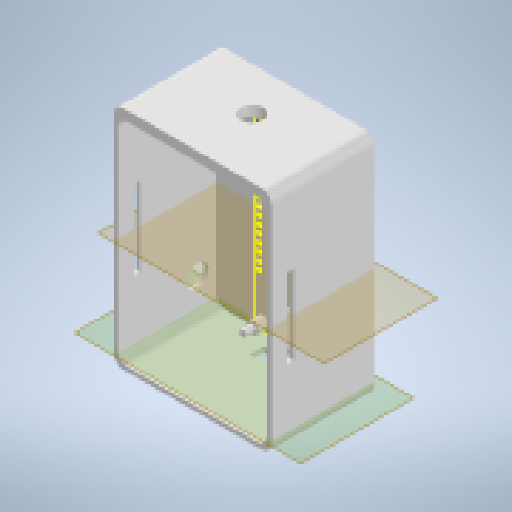
# Autodesk Inventor part: Casev2
Saved by Autodesk Inventor 2025.2 (Build 292293000, 293)
## iProperties
Created: 2022-04-07
Part Number: Casev2
Material: Generic
Document SubType Name: Modeling
Designer: Fred
Density: 1 g/cm^3
Appearance: Default
Author: Fred
## iProperties of the stored document CaseV2_3DPrint.ipt
Created: 2022-04-13
Part Number: CaseV2_3DPrint
Material: Generic
Document SubType Name: Modeling
Designer: Fred
Density: 1 g/cm^3
Appearance: Default
Author: Fred
Autodesk Inventor part; units mm, degrees
ref_plane "YZ Plane" through (0, 0, 0) normal (1, 0, 0) x (0, 1, 0)
ref_plane "XZ Plane" through (0, 0, 0) normal (0, 1, 0) x (-1, 0, 0)
sketch "Sketch1" plane through (0, 0, 0) normal (0, 0, 1) x (1, 0, 0)
  line L0 (0, 0) -> (50.8, 0)
  line L1 (50.8, 0) -> (50.8, 71.12)
  line L2 (50.8, 71.12) -> (0, 71.12)
  line L3 (0, 71.12) -> (0, 0)
  dimension "d0" = 71.12
  dimension "d1" = 50.8
  constraints: 8 end point, 2 parallel, 1 horizontal, 1 perpendicular
  measures "d0" distance of L0.end L1.end
  measures "d1" distance of L1.end L2.end
extrude "Extrusion1" add sketch "Sketch1" along normal blind 33
shell "Shell1" thickness 1.5 removed faces 1 at (33.8667, 23.7067, 33)
sketch "Sketch5" plane through (1.5, 69.62, 1.5) normal (0, 0, 1) x (1, 0, 0)
  circle A0 centre (15.01, -10.335) radius 1.1 projected
  circle A1 centre (15.01, -65.58) radius 1.25 projected
  circle A2 centre (32.79, -65.58) radius 1.25 projected
  circle A3 centre (13.74, -31.29) radius 0.6352 projected
  circle A4 centre (13.74, -23.67) radius 0.6352 projected
  circle A5 centre (34.06, -38.91) radius 0.6352 projected
  circle A6 centre (34.06, -41.45) radius 0.6352 projected
  circle A7 centre (34.06, -59.23) radius 0.6352 projected
  circle A8 centre (18.185, -32.544) radius 0.501 projected
  circle A9 centre (34.06, -31.29) radius 0.6352 projected
  circle A10 centre (13.74, -38.91) radius 0.6352 projected
  circle A11 centre (34.06, -54.15) radius 0.6352 projected
  circle A12 centre (34.06, -49.07) radius 0.6352 projected
  circle A13 centre (34.06, -23.67) radius 0.6352 projected
  circle A14 centre (13.74, -41.45) radius 0.6352 projected
  circle A15 centre (34.06, -28.75) radius 0.6352 projected
  circle A16 centre (13.74, -28.75) radius 0.6352 projected
  circle A17 centre (34.06, -26.21) radius 0.6352 projected
  circle A18 centre (34.06, -61.77) radius 0.6352 projected
  circle A19 centre (13.74, -51.61) radius 0.6352 projected
  circle A20 centre (34.06, -51.61) radius 0.6352 projected
  circle A21 centre (13.74, -49.07) radius 0.6352 projected
  circle A22 centre (34.06, -36.37) radius 0.6352 projected
  circle A23 centre (34.06, -46.53) radius 0.6352 projected
  circle A24 centre (34.06, -56.69) radius 0.6352 projected
  circle A25 centre (20.217, -30.544) radius 0.501 projected
  circle A26 centre (15.01, -10.335) radius 1.1 projected
  circle A27 centre (15.01, -65.58) radius 1.25 projected
  circle A28 centre (32.79, -65.58) radius 1.25 projected
  circle A29 centre (18.185, -30.544) radius 0.501 projected
  circle A30 centre (20.217, -32.544) radius 0.501 projected
  circle A31 centre (13.74, -36.37) radius 0.6352 projected
  circle A32 centre (34.06, -43.99) radius 0.6352 projected
  circle A33 centre (13.74, -33.83) radius 0.6352 projected
  circle A34 centre (13.74, -26.21) radius 0.6352 projected
  circle A35 centre (13.74, -46.53) radius 0.6352 projected
  circle A36 centre (34.06, -33.83) radius 0.6352 projected
  circle A37 centre (13.74, -43.99) radius 0.6352 projected
  line L0 (21.233, -68.12) -> (21.741, -67.612) projected
  line L1 (21.741, -67.612) -> (25.932, -67.612) projected
  line L2 (25.932, -67.612) -> (26.44, -68.12) projected
  line L3 (26.44, -68.12) -> (32.79, -68.12) projected
  arc A38 (32.79, -68.12) -> (35.33, -65.58) centre (32.79, -65.58) ccw projected
  line L4 (35.33, -65.58) -> (35.33, -10.335) projected
  arc A39 (35.33, -10.335) -> (32.79, -7.795) centre (32.79, -10.335) ccw projected
  line L5 (32.79, -7.795) -> (15.01, -7.795) projected
  arc A40 (15.01, -7.795) -> (12.47, -10.335) centre (15.01, -10.335) ccw projected
  line L6 (12.47, -10.335) -> (12.47, -65.58) projected
  arc A41 (12.47, -65.58) -> (15.01, -68.12) centre (15.01, -65.58) ccw projected
  line L7 (15.01, -68.12) -> (21.233, -68.12) projected
  point P0 (-1.5, -69.62)
  constraints: 3 coincident
ref_plane "Work Plane2" through (16.51, 4.04, 1.5) normal (0, -1, 0) x (1, 0, 0)
sketch "Sketch2" plane through (0, 71.12, 0) normal (0, 1, 0) x (1, 0, 0)
  line L0 (50.8, -33) -> (0, -33) projected
  line L1 (50.8, 0) -> (0, 0) projected
  point P0 (25.4, -13.95)
  point P1 (25.4, -13.95)
  point P2 (25.4, 0)
  dimension "d12" = 19.05
  constraints: 1 coincident, 1 midpoint, 1 vertical alignment
  measures "d12" distance from line of L0 point (25.4, -13.95)
hole "Hole1" at (25.4, 71.12, 13.95) direction (0, -1, 0) diameter 7.112 depth 1.5
thicken "Thicken1" operation add thickness 1.6 both sides no extend neighbours yes toward (0, 1, 0) faces at (25.4, 71.12, 27.8353)
ref_plane "Work Plane1" through (1.5, 35.56, 1.5) normal (0, 1, 0) x (1, 0, 0)
fillet "Fillet2" radius 3.175 8 edges at (0, 0, 16.5) (1.5, 1.5, 17.25) (1.5, 69.62, 17.25) (0, 72.72, 16.5) (50.8, 72.72, 16.5) (49.3, 69.62, 17.25) (50.8, 0, 16.5) (49.3, 1.5, 17.25)
sketch "Sketch6" plane through (3.175, 0, 0) normal (0, -1, 0) x (1, 0, 0)
  line L0 (19.264, 6.275) -> (18.264, 7.275) projected
  line L1 (25.064, 6.275) -> (19.264, 6.275) projected
  line L2 (26.064, 7.275) -> (25.064, 6.275) projected
  line L3 (26.064, 7.275) -> (26.064, 9.225) projected
  line L4 (18.264, 9.225) -> (26.064, 9.225) projected
  line L5 (18.264, 7.275) -> (18.264, 9.225) projected
  line L6 (17.502, 9.987) -> (26.826, 9.987)
  line L7 (26.826, 9.987) -> (26.826, 5.513)
  line L8 (26.826, 5.513) -> (17.502, 5.513)
  line L9 (17.502, 5.513) -> (17.502, 9.987)
  point P0 (-3.175, 0)
  dimension "d90" = 0.762
  dimension "d91" = 0.762
  dimension "d92" = 0.762
  dimension "d93" = 0.762
  constraints: 8 end point, 2 parallel, 1 horizontal, 1 perpendicular
  measures "d90" distance between parallel lines of L9 L5
  measures "d91" distance between parallel lines of L3 L7
  measures "d92" distance between parallel lines of L1 L8
  measures "d93" distance between parallel lines of L4 L6
extrude "Extrusion3" cut sketch "Sketch6" against normal blind 25.4 contours L0 L5 L4 L3 L2 L1 | L6 L7 L8 L9
chamfer "Chamfer1" distance 1.27 angle 45 1 edges at (25.339, 0, 9.987)
sketch "Sketch10" plane through (4.675, 69.62, 1.5) normal (0, 0, 1) x (1, 0, 0)
  circle A0 centre (10.465, -31.09) radius 0.6352 projected
  circle A1 centre (10.465, -23.47) radius 0.6352 projected
  circle A2 centre (30.785, -38.71) radius 0.6352 projected
  circle A3 centre (30.785, -41.25) radius 0.6352 projected
  circle A4 centre (30.785, -59.03) radius 0.6352 projected
  circle A5 centre (14.91, -32.344) radius 0.501 projected
  circle A6 centre (30.785, -31.09) radius 0.6352 projected
  circle A7 centre (10.465, -38.71) radius 0.6352 projected
  circle A8 centre (30.785, -53.95) radius 0.6352 projected
  circle A9 centre (30.785, -48.87) radius 0.6352 projected
  circle A10 centre (30.785, -23.47) radius 0.6352 projected
  circle A11 centre (10.465, -41.25) radius 0.6352 projected
  circle A12 centre (30.785, -28.55) radius 0.6352 projected
  circle A13 centre (10.465, -28.55) radius 0.6352 projected
  circle A14 centre (30.785, -26.01) radius 0.6352 projected
  circle A15 centre (30.785, -61.57) radius 0.6352 projected
  circle A16 centre (10.465, -51.41) radius 0.6352 projected
  circle A17 centre (30.785, -51.41) radius 0.6352 projected
  circle A18 centre (10.465, -48.87) radius 0.6352 projected
  circle A19 centre (30.785, -36.17) radius 0.6352 projected
  circle A20 centre (30.785, -46.33) radius 0.6352 projected
  circle A21 centre (30.785, -56.49) radius 0.6352 projected
  circle A22 centre (16.942, -30.344) radius 0.501 projected
  circle A23 centre (11.735, -65.38) radius 1.25 projected
  circle A24 centre (29.515, -65.38) radius 1.25 projected
  circle A25 centre (14.91, -30.344) radius 0.501 projected
  circle A26 centre (16.942, -32.344) radius 0.501 projected
  circle A27 centre (10.465, -36.17) radius 0.6352 projected
  circle A28 centre (30.785, -43.79) radius 0.6352 projected
  circle A29 centre (10.465, -33.63) radius 0.6352 projected
  circle A30 centre (10.465, -26.01) radius 0.6352 projected
  circle A31 centre (10.465, -46.33) radius 0.6352 projected
  circle A32 centre (30.785, -33.63) radius 0.6352 projected
  circle A33 centre (10.465, -43.79) radius 0.6352 projected
  line L0 (17.958, -67.92) -> (18.466, -67.412) projected
  line L1 (18.466, -67.412) -> (22.657, -67.412) projected
  line L2 (22.657, -67.412) -> (23.165, -67.92) projected
  line L3 (23.165, -67.92) -> (29.515, -67.92) projected
  arc A34 (29.515, -67.92) -> (32.055, -65.38) centre (29.515, -65.38) ccw projected
  line L4 (32.055, -65.38) -> (32.055, -10.135) projected
  arc A35 (32.055, -10.135) -> (29.515, -7.595) centre (29.515, -10.135) ccw projected
  line L5 (29.515, -7.595) -> (11.735, -7.595) projected
  arc A36 (11.735, -7.595) -> (9.195, -10.135) centre (11.735, -10.135) ccw
  line L6 (9.195, -10.135) -> (9.195, -65.38) projected
  arc A37 (9.195, -65.38) -> (11.735, -67.92) centre (11.735, -65.38) ccw projected
  line L7 (11.735, -67.92) -> (17.958, -67.92) projected
  circle A38 centre (10.465, -31.09) radius 0.6352 projected
  circle A39 centre (10.465, -23.47) radius 0.6352 projected
  circle A40 centre (30.785, -38.71) radius 0.6352 projected
  circle A41 centre (30.785, -41.25) radius 0.6352 projected
  circle A42 centre (30.785, -59.03) radius 0.6352 projected
  circle A43 centre (14.91, -32.344) radius 0.501 projected
  circle A44 centre (30.785, -31.09) radius 0.6352 projected
  circle A45 centre (10.465, -38.71) radius 0.6352 projected
  circle A46 centre (30.785, -53.95) radius 0.6352 projected
  circle A47 centre (30.785, -48.87) radius 0.6352 projected
  circle A48 centre (30.785, -23.47) radius 0.6352 projected
  circle A49 centre (10.465, -41.25) radius 0.6352 projected
  circle A50 centre (30.785, -28.55) radius 0.6352 projected
  circle A51 centre (10.465, -28.55) radius 0.6352 projected
  circle A52 centre (30.785, -26.01) radius 0.6352 projected
  circle A53 centre (30.785, -61.57) radius 0.6352 projected
  circle A54 centre (10.465, -51.41) radius 0.6352 projected
  circle A55 centre (30.785, -51.41) radius 0.6352 projected
  circle A56 centre (10.465, -48.87) radius 0.6352 projected
  circle A57 centre (30.785, -36.17) radius 0.6352 projected
  circle A58 centre (30.785, -46.33) radius 0.6352 projected
  circle A59 centre (30.785, -56.49) radius 0.6352 projected
  circle A60 centre (16.942, -30.344) radius 0.501 projected
  circle A61 centre (11.735, -65.38) radius 1.25 projected
  circle A62 centre (29.515, -65.38) radius 1.25 projected
  circle A63 centre (14.91, -30.344) radius 0.501 projected
  circle A64 centre (16.942, -32.344) radius 0.501 projected
  circle A65 centre (10.465, -36.17) radius 0.6352 projected
  circle A66 centre (30.785, -43.79) radius 0.6352 projected
  circle A67 centre (10.465, -33.63) radius 0.6352 projected
  circle A68 centre (10.465, -26.01) radius 0.6352 projected
  circle A69 centre (10.465, -46.33) radius 0.6352 projected
  circle A70 centre (30.785, -33.63) radius 0.6352 projected
  circle A71 centre (10.465, -43.79) radius 0.6352 projected
  line L8 (17.958, -67.92) -> (18.466, -67.412) projected
  line L9 (18.466, -67.412) -> (22.657, -67.412) projected
  line L10 (22.657, -67.412) -> (23.165, -67.92) projected
  line L11 (23.165, -67.92) -> (29.515, -67.92) projected
  arc A72 (29.515, -67.92) -> (32.055, -65.38) centre (29.515, -65.38) ccw projected
  line L12 (32.055, -65.38) -> (32.055, -10.135) projected
  arc A73 (32.055, -10.135) -> (29.515, -7.595) centre (29.515, -10.135) ccw projected
  line L13 (29.515, -7.595) -> (11.735, -7.595) projected
  arc A74 (11.735, -7.595) -> (9.195, -10.135) centre (11.735, -10.135) ccw
  line L14 (9.195, -10.135) -> (9.195, -65.38) projected
  arc A75 (9.195, -65.38) -> (11.735, -67.92) centre (11.735, -65.38) ccw projected
  line L15 (11.735, -67.92) -> (17.958, -67.92) projected
  circle A76 centre (11.735, -65.38) radius 1.905
  circle A77 centre (29.515, -65.38) radius 1.905
  circle A78 centre (11.735, -19.66) radius 1.905
  point P0 (-4.675, -69.62)
  dimension "d54" = 3.81
  dimension "d55" = 3.81
  dimension "d95" = 3.81
  dimension "d96" = 45.72
  constraints: 5 centre point, 4 point on circle, 2 coincident, 1 vertical alignment
  measures "d54" diameter of A76
  measures "d55" diameter of A77
  measures "d95" diameter of A78
  measures "d96" distance of A75.centre A78.centre
ref_plane "Work Plane4" through (21.59, 1.6, 4.775) normal (0, 0, -1) x (0, 1, 0)
extrude "Extrusion7" add sketch "Sketch10" along normal up to surface (3.275 mm away) contours A23 | A24 | A76 | A77 | A78
sketch "Sketch11" plane through (34.19, 4.24, 4.775) normal (0, 0, 1) x (1, 0, 0)
  circle A0 centre (0, 0) radius 1.016
  circle A1 centre (-17.78, 0) radius 1.905 projected
  circle A2 centre (-17.78, 0) radius 1.016
  circle A3 centre (-17.78, 45.72) radius 1.905 projected
  circle A4 centre (-17.78, 45.72) radius 1.905 projected
  circle A5 centre (-17.78, 45.72) radius 1.016
  point P0 (-34.19, -4.24)
  point P1 (-17.78, 55.245)
  dimension "d59" = 2.032
  dimension "d60" = 2.032
  dimension "d97" = 2.032
  constraints: 3 centre point, 2 coincident
  measures "d59" diameter of A0
  measures "d60" diameter of A2
  measures "d97" diameter of A5
extrude "Extrusion8" add sketch "Sketch11" along normal blind 3.175 contours A0 | A2 | A5
sketch "Sketch13" plane through (4.675, 69.62, 1.5) normal (0, 0, 1) x (1, 0, 0)
  line L0 (44.625, -16.28) -> (36.751, -16.28)
  line L1 (36.751, -16.28) -> (36.751, -51.84)
  line L2 (36.751, -51.84) -> (44.625, -51.84)
  line L3 (44.625, -51.84) -> (44.625, -16.28)
  line L4 (44.625, -3.175) -> (44.625, -64.945) projected
  line L5 (45.895, -15.01) -> (35.481, -15.01)
  line L6 (35.481, -15.01) -> (35.481, -53.11)
  line L7 (35.481, -53.11) -> (45.895, -53.11)
  line L8 (45.895, -53.11) -> (45.895, -15.01)
  point P0 (-4.675, -69.62)
  point P1 (44.625, -34.06)
  point P2 (44.625, -34.06)
  dimension "d72" = 35.56
  dimension "d73" = 7.874
  dimension "d74" = 0
  dimension "d75" = 1.27
  constraints: 16 end point, 4 parallel, 2 midpoint, 2 perpendicular, 1 coincident, 1 horizontal, 3 other
  measures "d72" distance of L2.end L0.start
  measures "d73" distance of L0.start L0.end
  measures "d74" distance between parallel lines of L4 L3
  measures "d75" distance between parallel lines of L3 L8
extrude "Extrusion10" add sketch "Sketch13" along normal blind 17.018 contours L4 L5 L8 L7 L3 | L0 L1 L2 L4 L7 L6 L5
sketch "Sketch14" plane through (4.675, 69.62, 18.518) normal (0, 0, 1) x (1, 0, 0)
  line L0 (40.615, -14.91) -> (40.615, -53.01) projected
  line L1 (35.481, -53.11) -> (35.481, -15.01) projected
  line L2 (41.885, -41.68) -> (34.211, -41.68)
  line L3 (34.211, -41.68) -> (34.211, -26.44)
  line L4 (34.211, -26.44) -> (41.885, -26.44)
  line L5 (41.885, -26.44) -> (41.885, -41.68)
  line L6 (36.751, -16.28) -> (44.625, -16.28) projected
  line L7 (44.625, -51.84) -> (36.751, -51.84) projected
  point P0 (-4.675, -69.62)
  point P1 (40.615, -26.44)
  point P2 (35.481, -26.44)
  point P3 (35.481, -41.68)
  point P4 (40.615, -41.68)
  dimension "d78" = 10.16
  dimension "d79" = 10.16
  dimension "d88" = 1.27
  dimension "d89" = 1.27
  constraints: 8 end point, 2 parallel, 1 horizontal, 1 perpendicular
  measures "d78" distance between parallel lines of L6 L4
  measures "d79" distance between parallel lines of L7 L2
  measures "d88" distance between parallel lines of L3 L1
  measures "d89" distance between parallel lines of L0 L5
extrude "Extrusion11" cut sketch "Sketch14" against normal up to surface (17.018 mm away) contours L0 L2 L1 L4
fillet "Fillet6" radius 1.27 2 edges at (40.156, 54.61, 10.009) (40.156, 16.51, 10.009)
sketch "Sketch15" plane through (0, 3.175, 0) normal (-1, 0, 0) x (0, 0, 1)
  line L0 (28, 45.085) -> (26, 45.085)
  line L1 (26, 45.085) -> (26, 19.685)
  line L2 (26, 19.685) -> (28, 19.685)
  line L3 (28, 19.685) -> (28, 45.085)
  line L4 (33, 1.5) -> (33, 63.27) projected
  point P0 (0, -3.175)
  point P1 (26, 32.385)
  point P2 (33, 32.385)
  dimension "d83" = 25.4
  dimension "d84" = 2
  dimension "d85" = 7
  constraints: 8 end point, 2 midpoint, 2 parallel, 1 horizontal, 1 horizontal alignment, 1 perpendicular
  measures "d83" distance of L0.end L1.end
  measures "d84" distance of L0.start L0.end
  measures "d85" distance between parallel lines of L4 L1
extrude "Extrusion12" cut sketch "Sketch15" against normal through all
sketch "Sketch16" plane through (0, 3.175, 0) normal (-1, 0, 0) x (0, 0, 1)
  circle A0 centre (7.62, 9.525) radius 3.556
  line L0 (0, -3.175) -> (33, -3.175) projected
  line L1 (0, 66.37) -> (0, 0) projected
  dimension "d98" = 7.112
  dimension "d99" = 12.7
  dimension "d100" = 7.62
  constraints: 1 centre point
  measures "d98" diameter of A0
  measures "d99" distance from line of L0 A0.centre
  measures "d100" distance from line of L1 A0.centre
extrude "Extrusion13" cut sketch "Sketch16" against normal up to surface (1.5 mm away)
equation "\"d55\" = d54"
equation "\"d60\" = d59"
body "Solid1"
